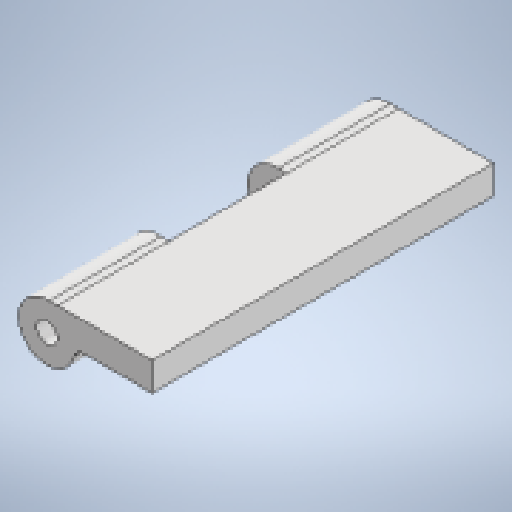
# Autodesk Inventor part: outerhinge
Saved by Autodesk Inventor 2026 (Build 300175050, 175E)
## iProperties
Created: 2025-10-10
Part Number: outerhinge
Material: Generic
Document SubType Name: Modeling
Designer: Nicholas M
Density: 1 g/cm^3
Appearance: Default
Author: Nicholas M
Autodesk Inventor part; units mm, degrees
ref_plane "YZ Plane" through (0, 0, 0) normal (1, 0, 0) x (0, 1, 0)
ref_plane "XZ Plane" through (0, 0, 0) normal (0, 1, 0) x (-1, 0, 0)
ref_plane "XY Plane" through (0, 0, 0) normal (0, 0, 1) x (1, 0, 0)
sketch "Sketch1" plane through (0, 0, 0) normal (0, 0, 1) x (1, 0, 0)
  circle A0 centre (0, 0) radius 0.6985
  circle A1 centre (0, 0) radius 1.905
  line L0 (0.6985, 0) -> (7.0485, 0)
  line L1 (7.0485, 0) -> (7.0485, 1.905)
  line L2 (7.0485, 1.905) -> (0.6985, 1.905)
  line L3 (0.6985, 1.905) -> (0.6985, 0)
  point P0 (0.6985, 1.7723)
  point P1 (1.905, 0)
  dimension "d0" = 1.397
  dimension "d1" = 3.81
  dimension "d4" = 6.35
  dimension "d5" = 1.905
  constraints: 8 end point, 2 coincident, 2 horizontal alignment, 2 parallel, 1 centre point, 1 horizontal, 1 perpendicular, 2 other
  measures "d1" diameter of A1
  measures "d4" distance of L2.end L1.end
  measures "d5" distance of L1.end L0.end
extrude "Extrusion1" add sketch "Sketch1" along normal blind 7.493
fillet "Fillet1" radius 3.175 1 edges at (0.6985, 1.7723, 3.7465)
fillet "Fillet2" radius 0.5292 1 edges at (1.905, 0, 3.7465)
sketch "Sketch2" plane through (0, 0, 0) normal (0, 0, -1) x (-1, 0, 0)
  arc A0 (-0.6985, 1.905) -> (-0.1463, 1.8994) centre (-0.3902, 5.065) ccw projected
  line L0 (-7.0485, 1.905) -> (-0.6985, 1.905) projected
  line L1 (-7.0485, 0) -> (-7.0485, 1.905) projected
  line L2 (-2.376, 0) -> (-7.0485, 0) projected
  arc A1 (-1.8594, -0.4141) -> (-2.376, 0) centre (-2.376, -0.5292) ccw projected
  arc A2 (-1.8594, -0.4141) -> (-0.1463, 1.8994) centre (0, 0) ccw projected
  circle A3 centre (0, 0) radius 0.6985 projected
  circle A4 centre (0, 0) radius 1.905
  circle A5 centre (0, 0) radius 2.032
  line L3 (-0.5019, 1.969) -> (-0.5019, 1.892)
  point P0 (-2.0278, -0.1307)
  point P1 (0.0205, 1.3968)
  point P2 (-0.7071, 1.905)
  dimension "d8" = 0.127
  constraints: 2 end point, 1 centre point, 1 coincident, 1 concentric, 1 point on circle, 1 vertical, 3 other
extrude "Extrusion2" add sketch "Sketch2" along normal blind 7.874 contours A5 A1 L2 L1 L0
extrude "Extrusion3" add sketch "Sketch2" along normal blind 7.493 from surface at 7.874 contours A0 A4 A1 A5 L0 | A5 A1 L2 L1 L0 | A2 A4
body "Solid1"
